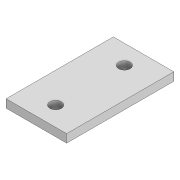
# Autodesk Inventor part: 90 graders beslag
Saved by Autodesk Inventor 2021 (Build 250183000, 183)
## iProperties
Created: 2020-11-05
Part Number: 90 graders beslag
Material: Generic
Document SubType Name: Sheet Metal
Designer: Alfred Brauner
Density: 1 g/cm^3
Sheet Metal Rule: Default_mm
Appearance: Default
Author: Alfred Brauner
Autodesk Inventor part; units mm, degrees
ref_plane "YZ Plane" through (0, 0, 0) normal (1, 0, 0) x (0, 1, 0)
ref_plane "XZ Plane" through (0, 0, 0) normal (0, 1, 0) x (-1, 0, 0)
ref_plane "XY Plane" through (0, 0, 0) normal (0, 0, 1) x (1, 0, 0)
sketch "Sketch1" plane through (0, 0, 0) normal (0, 1, 0) x (-1, 0, 0)
  line L0 (11, 19.5) -> (-11, 19.5)
  line L1 (-11, 19.5) -> (-11, -19.5)
  line L2 (-11, -19.5) -> (11, -19.5)
  line L3 (11, -19.5) -> (11, 19.5)
  line L4 (11, 19.5) -> (-11, -19.5) construction
  line L5 (-11, 19.5) -> (11, -19.5) construction
  point P0 (0, 0)
  dimension "d0" = 22
  dimension "d1" = 39
  measures "d0" distance of L2.end L1.end
  measures "d1" distance of L1.end L0.end
extrude "Plate1" add sketch "Sketch1" along normal blind 3
sketch "Sketch2" plane through (0, 3, 0) normal (0, 1, 0) x (1, 0, 0)
  circle A0 centre (0, -12.5) radius 2.1
  line L0 (11, -19.5) -> (11, 19.5) projected
  line L1 (11, 0) -> (-11, 0)
  line L2 (-11, 19.5) -> (-11, -19.5) projected
  circle A1 centre (0, 12.5) radius 2.1
  point P0 (0, 0)
  dimension "d3" = 4.2
  dimension "d4" = 12.5
  constraints: 2 centre point, 2 end point, 2 midpoint, 1 symmetric about line, 1 other
  measures "d3" diameter of A0
  measures "d4" distance of point (0, 0) A0.centre
extrude "Cut1" cut sketch "Sketch2" against normal blind 3
equation "\"d5\" = Thickness"
equation "\"d2\" = Thickness"
equation "\"BendRadius\" = Thickness"
equation "\"BendReliefWidth\" = Thickness"
equation "\"BendReliefDepth\" = 0.5 * Thickness"
equation "\"CornerReliefSize\" = 4 * Thickness"
equation "\"MinimumRemnant\" = 2 * Thickness"
equation "\"TransitionRadius\" = BendRadius"
equation "\"JacobiRadiusSize\" = BendRadius"
equation "\"GapSize\" = Thickness"
equation "\"Thickness\" = 3"
body "Solid1"
